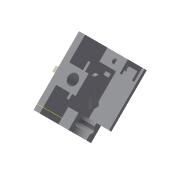
# Autodesk Inventor part: OPENTRONS_autofocus_astigmatism_base
Saved by Autodesk Inventor 2019.4 (Build 234330000, 330)
## iProperties
Created: 2021-01-25
Part Number: OPENTRONS_autofocus_astigmatism_base
Material: Generic
Document SubType Name: Modeling
Designer: diederichbenedict
Density: 1 g/cm^3
Appearance: Default
Author: diederichbenedict
Autodesk Inventor part; units mm, degrees
ref_plane "YZ Plane" through (0, 0, 0) normal (1, 0, 0) x (0, 1, 0)
ref_plane "Work Plane1" through (-9, 9, -0.2) normal (-1, 0, 0) x (0, 0, 1)
ref_plane "Work Plane2" through (-10.673, 19.085, 18.1993) normal (-1, 0, 0) x (0, -0.7071068, -0.7071068)
sketch "Sketch1" plane through (-10.673, 19.085, 18.1993) normal (-1, 0, 0) x (0, -0.7071068, -0.7071068)
  line L0 (22.0054, -17.7377) -> (31.0054, -17.7377) projected
  line L1 (22.0054, -17.7377) -> (22.0054, -15.7377) projected
  line L2 (31.0054, -15.7377) -> (22.0054, -15.7377) projected
  line L3 (31.0054, -17.7377) -> (31.0054, -15.7377) projected
  line L4 (37.2508, -20.2498) -> (-0.7492, -20.2498)
  line L5 (-0.7492, -20.2498) -> (-0.7492, 21.7502)
  line L6 (-0.7492, 21.7502) -> (37.2508, 21.7502)
  line L7 (37.2508, 21.7502) -> (37.2508, -20.2498)
  point P0 (26.364, 0.6263)
  dimension "d0" = 38
  dimension "d1" = 42
  constraints: 8 end point, 2 parallel, 1 horizontal, 1 perpendicular
  measures "d0" distance of L5.end L6.end
  measures "d1" distance of L4.end L5.end
extrude "Extrusion1" add sketch "Sketch1" against normal blind 4 contours L1 L2 L3 L0 | L4 L5 L6 L7
sketch "Sketch2" plane through (-10.673, 4.235, 34.1088) normal (0, 0.7071068, 0.7071068) x (1, 0, 0)
  circle A0 centre (10.673, 21.2654) radius 3 projected
  line L0 (4, 42) -> (4, 0) projected
  line L1 (4, 27.2654) -> (16.673, 27.2654)
  line L2 (16.673, 27.2654) -> (16.673, 15.2654)
  line L3 (16.673, 15.2654) -> (4, 15.2654)
  line L4 (4, 15.2654) -> (4, 27.2654)
  circle A1 centre (10.673, 21.2654) radius 3.3
  point P0 (10.673, 21.1239)
  dimension "d4" = 6
  dimension "d5" = 6
  dimension "d6" = 6
  dimension "d7" = 0.3
  constraints: 8 end point, 2 parallel, 1 centre point, 1 horizontal, 1 perpendicular, 1 point on line
  measures "d4" distance from line of A0.centre L1
  measures "d5" distance from line of L3 A0.centre
  measures "d6" distance from line of L2 A0.centre
  measures "d7" radial gap between concentric circles of A0 A1
ref_plane "Work Plane3" through (-3, 11.6711, 11.4711) normal (0, -0.7071068, -0.7071068) x (1, 0, 0)
extrude "Extrusion2" add sketch "Sketch2" against normal up to surface (10.7492 mm away) contours L1 L2 L3 L0
sketch "Sketch3" plane through (-6.673, 19.085, 18.1993) normal (1, 0, 0) x (0, 0.7071068, -0.7071068)
  line L0 (-6.9903, -32.7279) -> (5.7377, -20) projected
  line L1 (-6.8488, -32.8693) -> (5.8791, -20.1414) projected
  line L2 (5.6912, -19.9536) -> (-7.0367, -32.6815)
  line L3 (-7.0367, -32.6815) -> (-8.4509, -31.2673)
  line L4 (-8.4509, -31.2673) -> (4.277, -18.5393)
  line L5 (4.277, -18.5393) -> (5.6912, -19.9536)
  line L6 (-6.7535, -32.9646) -> (5.9323, -20.1947)
  line L7 (5.9323, -20.1947) -> (7.3512, -21.6042)
  line L8 (7.3512, -21.6042) -> (-5.3347, -34.3742)
  line L9 (-5.3347, -34.3742) -> (-6.7535, -32.9646)
  point P0 (-0.6263, -26.364)
  dimension "d10" = 2
  dimension "d11" = 2
  constraints: 16 end point, 5 parallel, 2 perpendicular, 2 point on line
  measures "d10" distance of L2.end L3.end
  measures "d11" distance of L6.end L7.end
sketch "Sketch4" plane through (-6.673, 33.9335, 4.4103) normal (0, 0.7071068, -0.7071068) x (-1, 0, 0)
  line L0 (4, -38) -> (4, 0) projected
  line L1 (4, 0) -> (0, 0) projected
  line L2 (0, -38) -> (0, 0) projected
  line L3 (4, -38) -> (0, -38) projected
  line L4 (-2.173, -31.7546) -> (-2.173, -22.7546) projected
  line L5 (-2.173, -22.7546) -> (-11.173, -22.7546) projected
  line L6 (-11.173, -22.7546) -> (-11.173, -31.7546) projected
  line L7 (-11.173, -31.7546) -> (-2.173, -31.7546) projected
  line L8 (-1.873, -22.4546) -> (-1.873, -32.0546)
  line L9 (-1.873, -32.0546) -> (-11.473, -32.0546)
  line L10 (-11.473, -32.0546) -> (-11.473, -22.4546)
  line L11 (-11.473, -22.4546) -> (-1.873, -22.4546)
  line L12 (0, -33.9276) -> (0, -20.5815)
  line L13 (0, -20.5815) -> (-13.3461, -20.5815)
  line L14 (-13.3461, -20.5815) -> (-13.3461, -33.9276)
  line L15 (-13.3461, -33.9276) -> (0, -33.9276)
  point P0 (-6.673, -27.1131)
  dimension "d12" = 0.3
  constraints: 16 end point, 1 point on line, 6 other
  measures "d12" distance between parallel lines of L4 L8
ref_plane "Work Plane4" through (-4.5, 9.7033, -16.2673) normal (0, 0.7071068, -0.7071068) x (0, 0.7071068, 0.7071068)
extrude "Extrusion3" add sketch "Sketch4" against normal up to surface (2.5121 mm away) contours L15 L14 L13 L2 | L7 L6 L5 L4 | L8 L9 L10 L11
sketch "Sketch5" plane through (6.673, 9.943, -19.5802) normal (1, 0, 0) x (0, 0.7071068, -0.7071068)
  line L0 (-2.5121, 0) -> (-2.5121, 13.3461) projected
  line L1 (0, 0) -> (-2.5121, 0) projected
  line L2 (0, 0) -> (0, 13.3461) projected
  line L3 (0, 13.3461) -> (-2.5121, 13.3461) projected
  line L4 (-2.5121, 2.173) -> (-4.5121, 2.173) projected
  line L5 (-2.5121, 11.173) -> (-4.5121, 11.173) projected
  line L6 (0, 0) -> (-2.5121, 0) projected
  line L7 (-2.5121, 0) -> (-7.5121, 0)
  line L8 (-7.5121, 0) -> (-7.5121, 2)
  line L9 (-7.5121, 2) -> (-2.5121, 2)
  line L10 (-2.5121, 2) -> (-2.5121, 0)
  line L11 (-2.5121, 13.3461) -> (-7.5121, 13.3461)
  line L12 (-7.5121, 13.3461) -> (-7.5121, 11.3461)
  line L13 (-7.5121, 11.3461) -> (-2.5121, 11.3461)
  line L14 (-2.5121, 11.3461) -> (-2.5121, 13.3461)
  point P0 (-20.8761, 6.8145)
  dimension "d15" = 5
  dimension "d16" = 2
  dimension "d17" = 5
  dimension "d18" = 2
  constraints: 16 end point, 4 parallel, 2 horizontal, 2 perpendicular
  measures "d15" distance of L8.end L9.end
  measures "d16" distance of L7.end L8.end
  measures "d17" distance of L13.end L12.end
  measures "d18" distance of L12.end L11.end
extrude "Extrusion4" add sketch "Sketch5" against normal up to surface (13.3461 mm away) contours L7 L8 L9 L0 | L0 L13 L12 L11
sketch "Sketch6" plane through (-6.673, 19.3802, -10.143) normal (0, 0.7071068, 0.7071068) x (1, 0, 0)
  line L0 (11.173, -4.5121) -> (2.173, -4.5121) projected
  circle A0 centre (7.5134, -3.8582) radius 1.45
  point P0 (6.673, -20.8761)
  dimension "d21" = 2.9
  constraints: 1 centre point
  measures "d21" diameter of A0
extrude "Extrusion5" cut sketch "Sketch6" against normal through all
extrude "Extrusion6" add sketch "Sketch3" along normal blind 2
ref_plane "Work Plane5" through (-10.673, -20.337, 4.9406) normal (0, -0.7071068, 0.7071068) x (1, 0, 0)
sketch "Sketch7" plane through (-10.673, -20.337, 4.9406) normal (0, -0.7071068, 0.7071068) x (1, 0, 0)
  circle A0 centre (10.673, 10.7454) radius 7.86 projected
  circle A1 centre (10.673, 10.7454) radius 6.9153
  line L0 (4, 0) -> (4, 4.0724) projected
  line L1 (4, 0) -> (10.673, 0)
  line L2 (10.673, 0) -> (10.673, 20.7944)
  line L3 (10.673, 20.7944) -> (4, 20.7944)
  line L4 (4, 20.7944) -> (4, 0)
  point P0 (10.673, 10.8869)
  point P1 (10.673, 17.6608)
  point P2 (10.673, 3.8301)
  constraints: 8 end point, 3 point on line, 2 parallel, 2 point on circle, 1 centre point, 1 horizontal, 1 perpendicular
extrude "Extrusion7" add sketch "Sketch7" along normal blind 3.25 and the other way blind 6 contours L2 A1 L4 A0 | A0 L4 L3 L2 | L2 L1 L0 L4 A0 | A0 L4 A1 L2 | L2 A1 L4
sketch "Sketch8" plane through (0, -22.6351, 7.2387) normal (1, 0, 0) x (0, 0.7071068, -0.7071068)
  line L0 (5.4879, 2.8854) -> (4.4879, 2.8854)
  arc A0 (7.4621, 17.2093) -> (5.5461, 18.8054) centre (0.4542, 10.7454) ccw
  line L1 (5.5461, 2.6854) -> (4.3934, 2.6854)
  arc A1 (4.3934, 18.8054) -> (3.267, 17.2093) centre (14.12, 10.7454) ccw
  line L2 (4.3934, 18.8054) -> (5.5461, 18.8054)
  line L3 (7.4621, 17.2093) -> (12.254, 17.2093)
  line L4 (12.254, 17.2093) -> (12.254, 10.7454)
  line L5 (12.254, 10.7454) -> (-1.0858, 10.7454)
  line L6 (-1.0858, 10.7454) -> (-1.0858, 17.2093)
  line L7 (-1.0858, 17.2093) -> (3.267, 17.2093)
  point P0 (21.1239, 10.8869)
  point P1 (9.7879, 10.7454)
  point P2 (1.6341, 10.7454)
  point P3 (1.6879, 10.7454)
  point P4 (1.4879, 10.7454)
  point P5 (9.9879, 10.7454)
  constraints: 16 end point, 7 point on line, 4 point on circle, 3 perpendicular, 2 centre point, 2 horizontal, 4 other
revolve "Revolution1" cut sketch "Sketch8" angle 360 about axis through (0, -6.372, 6.172) along (0, -0.7071068, 0.7071068)
sketch "Sketch9" plane through (-6.673, 19.085, 18.1993) normal (1, 0, 0) x (0, 0.7071068, -0.7071068)
  line L0 (-21.7502, -16.4565) -> (-12.5002, -16.4565) projected
  line L1 (-12.5002, -16.4565) -> (-12.5002, -37.2508) projected
  line L2 (-12.5002, -37.2508) -> (20.2498, -37.2508) projected
  line L3 (20.2498, -37.2508) -> (20.2498, -33.1784) projected
  line L4 (20.2498, -33.1784) -> (12.7377, -33.1784) projected
  line L5 (12.7377, -33.1784) -> (12.7377, -31.1784) projected
  line L6 (12.7377, -31.1784) -> (17.7377, -31.1784) projected
  line L7 (17.7377, -31.1784) -> (17.7377, -21.8323) projected
  line L8 (17.7377, -21.8323) -> (12.7377, -21.8323) projected
  line L9 (12.7377, -21.8323) -> (12.7377, -19.8323) projected
  line L10 (12.7377, -19.8323) -> (20.2498, -19.8323) projected
  line L11 (20.2498, -19.8323) -> (20.2498, 0.7492) projected
  line L12 (20.2498, 0.7492) -> (5.5151, 0.7492) projected
  line L13 (5.5151, 0.7492) -> (5.5151, -10) projected
  line L14 (5.5151, -10) -> (-6.4849, -10) projected
  line L15 (-6.4849, -10) -> (-6.4849, 0.7492) projected
  line L16 (-6.4849, 0.7492) -> (-21.7502, 0.7492) projected
  line L17 (-21.7502, 0.7492) -> (-21.7502, -16.4565) projected
  line L18 (5.9323, -20.1947) -> (7.3512, -21.6042) projected
  line L19 (7.3512, -21.6042) -> (-5.3347, -34.3742) projected
  line L20 (-5.3347, -34.3742) -> (-6.7535, -32.9646) projected
  line L21 (-6.7535, -32.9646) -> (5.9323, -20.1947) projected
  line L22 (-7.0367, -32.6815) -> (-8.4509, -31.2673) projected
  line L23 (-8.4509, -31.2673) -> (4.277, -18.5393) projected
  line L24 (4.277, -18.5393) -> (5.6912, -19.9536) projected
  line L25 (5.6912, -19.9536) -> (-7.0367, -32.6815) projected
  line L26 (-12.5002, -16.4565) -> (-12.5002, -37.2508) projected
  line L27 (-12.5002, -37.2508) -> (20.2498, -37.2508)
  line L28 (20.2498, -37.2508) -> (20.2498, -35.2508)
  line L29 (20.2498, -35.2508) -> (-12.5002, -35.2508)
  line L30 (-12.5002, -35.2508) -> (-12.5002, -37.2508)
  point P0 (-0.6263, -26.364)
  dimension "d33" = 2
  constraints: 8 end point, 2 parallel, 1 horizontal, 1 perpendicular, 1 point on line
  measures "d33" distance of L28.end L27.end
extrude "Extrusion8" add sketch "Sketch9" along normal up to surface (13.3461 mm away) contours L29 L3 L2 L1
sketch "Sketch10" plane through (-6.673, 19.085, 18.1993) normal (1, 0, 0) x (0, 0.7071068, -0.7071068)
  line L0 (-12.5002, -35.2508) -> (20.2498, -35.2508) projected
  line L1 (20.2498, -35.2508) -> (20.2498, -33.1784) projected
  line L2 (20.2498, -33.1784) -> (12.7377, -33.1784) projected
  line L3 (12.7377, -33.1784) -> (12.7377, -31.1784) projected
  line L4 (12.7377, -31.1784) -> (17.7377, -31.1784) projected
  line L5 (17.7377, -31.1784) -> (17.7377, -21.8323) projected
  line L6 (17.7377, -21.8323) -> (12.7377, -21.8323) projected
  line L7 (12.7377, -21.8323) -> (12.7377, -19.8323) projected
  line L8 (12.7377, -19.8323) -> (20.2498, -19.8323) projected
  line L9 (20.2498, -19.8323) -> (20.2498, 0.7492) projected
  line L10 (20.2498, 0.7492) -> (5.5151, 0.7492) projected
  line L11 (5.5151, 0.7492) -> (5.5151, -10) projected
  line L12 (5.5151, -10) -> (-6.4849, -10) projected
  line L13 (-6.4849, -10) -> (-6.4849, 0.7492) projected
  line L14 (-6.4849, 0.7492) -> (-21.7502, 0.7492) projected
  line L15 (-21.7502, 0.7492) -> (-21.7502, -16.4565) projected
  line L16 (-21.7502, -16.4565) -> (-12.5002, -16.4565) projected
  line L17 (-12.5002, -16.4565) -> (-12.5002, -35.2508) projected
  line L18 (5.9323, -20.1947) -> (7.3512, -21.6042) projected
  line L19 (7.3512, -21.6042) -> (-5.3347, -34.3742) projected
  line L20 (-5.3347, -34.3742) -> (-6.7535, -32.9646) projected
  line L21 (-6.7535, -32.9646) -> (5.9323, -20.1947) projected
  line L22 (-7.0367, -32.6815) -> (-8.4509, -31.2673) projected
  line L23 (-8.4509, -31.2673) -> (4.277, -18.5393) projected
  line L24 (4.277, -18.5393) -> (5.6912, -19.9536) projected
  line L25 (5.6912, -19.9536) -> (-7.0367, -32.6815) projected
  line L26 (5.6912, -19.9536) -> (-7.0367, -32.6815) projected
  line L27 (5.6912, -19.9536) -> (5.9323, -20.1947)
  line L28 (5.9323, -20.1947) -> (-6.7956, -32.9226)
  line L29 (-6.7956, -32.9226) -> (-7.0367, -32.6815)
  line L30 (-7.0367, -32.6815) -> (5.6912, -19.9536)
  line L31 (-9.5283, -11.9065) -> (10.4717, -11.9065)
  line L32 (10.4717, -11.9065) -> (10.4717, -13.9065)
  line L33 (10.4717, -13.9065) -> (-9.5283, -13.9065)
  line L34 (-9.5283, -13.9065) -> (-9.5283, -11.9065)
  line L35 (10.4717, -22.6297) -> (10.4717, -32.6297)
  line L36 (10.4717, -32.6297) -> (8.4717, -32.6297)
  line L37 (8.4717, -32.6297) -> (8.4717, -22.6297)
  line L38 (8.4717, -22.6297) -> (10.4717, -22.6297)
  point P0 (-0.6263, -26.364)
  dimension "d36" = 20
  dimension "d37" = 2
  dimension "d40" = 10
  dimension "d41" = 2
  constraints: 24 end point, 6 parallel, 4 perpendicular, 1 horizontal, 1 vertical
  measures "d36" distance of L31.start L31.end
  measures "d37" distance of L31.end L32.end
  measures "d40" distance of L35.start L35.end
  measures "d41" distance of L35.end L36.end
extrude "Extrusion9" cut sketch "Sketch10" against normal blind 3.25 contours L28 L29 L25 L27 | L31 L32 L33 L34 | L35 L36 L37 L38
body "Solid1"
